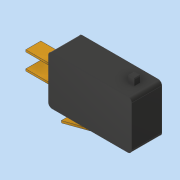
# Autodesk Inventor part: LIMIT SWITCH
Saved by Autodesk Inventor 2017 (Build 210142000, 142)
## iProperties
Created: 2016-02-15
Part Number: LIMIT SWITCH
Material: Generic
Document SubType Name: Modeling
Designer: techn
Density: 1 g/cm^3
Appearance: Smooth - Black
Author: techn
Autodesk Inventor part; units mm, degrees
ref_plane "YZ Plane" through (0, 0, 0) normal (1, 0, 0) x (0, 1, 0)
ref_plane "XZ Plane" through (0, 0, 0) normal (0, 1, 0) x (-1, 0, 0)
ref_plane "XY Plane" through (0, 0, 0) normal (0, 0, 1) x (1, 0, 0)
sketch "Sketch1" plane through (0, 0, 0) normal (0, 0, 1) x (1, 0, 0)
  line L0 (0, 0) -> (27.94, 0)
  line L1 (27.94, 0) -> (27.94, 16.256)
  line L2 (27.94, 16.256) -> (0, 16.256)
  line L3 (0, 16.256) -> (0, 0)
  dimension "d0" = 27.94
  dimension "d1" = 16.256
  constraints: 8 end point, 2 parallel, 1 horizontal, 1 perpendicular
  measures "d0" distance of L2.end L1.end
  measures "d1" distance of L1.end L0.end
extrude "Extrusion1" add sketch "Sketch1" along normal blind 10.16
fillet "Fillet1" radius 1.27 4 edges at (0, 16.256, 5.08) (27.94, 16.256, 5.08) (27.94, 0, 5.08) (0, 0, 5.08)
sketch "Sketch3" plane through (0, 0, 10.16) normal (0, 0, 1) x (1, 0, 0)
  arc A0 (0, 1.27) -> (1.27, 0) centre (1.27, 1.27) ccw projected
  line L0 (1.27, 0) -> (26.67, 0) projected
  arc A1 (26.67, 0) -> (27.94, 1.27) centre (26.67, 1.27) ccw projected
  line L1 (27.94, 1.27) -> (27.94, 14.986) projected
  arc A2 (27.94, 14.986) -> (26.67, 16.256) centre (26.67, 14.986) ccw projected
  line L2 (26.67, 16.256) -> (1.27, 16.256) projected
  arc A3 (1.27, 16.256) -> (0, 14.986) centre (1.27, 14.986) ccw projected
  line L3 (0, 14.986) -> (0, 1.27) projected
  line L4 (26.67, 16.256) -> (1.27, 16.256) projected
  line L5 (24.765, 16.256) -> (24.765, 18.542)
  line L6 (24.765, 18.542) -> (22.733, 18.542)
  line L7 (22.733, 18.542) -> (22.733, 16.256)
  point P0 (0, 0)
  dimension "d12" = 2.286
  dimension "d13" = 2.032
  dimension "d14" = 3.175
  constraints: 6 end point, 2 perpendicular, 2 point on line, 1 horizontal
  measures "d12" distance of L5.start L5.end
  measures "d13" distance of L5.end L6.end
  measures "d14" distance between parallel lines of L1 L5
ref_plane "Work Plane1" through (0, 0, 5.08) normal (0, 0, 1) x (1, 0, 0)
sketch "Sketch4" plane through (0, 0, 5.08) normal (0, 0, 1) x (1, 0, 0)
  line L0 (24.765, 18.542) -> (22.733, 18.542) projected
  line L1 (22.733, 18.542) -> (22.733, 16.256) projected
  line L2 (24.765, 16.256) -> (24.765, 18.542) projected
  line L3 (22.733, 16.256) -> (24.765, 16.256)
  line L4 (26.67, 16.256) -> (1.27, 16.256) projected
  point P0 (0, 0)
  constraints: 2 end point, 1 collinear
extrude "Extrusion3" add sketch "Sketch4" along normal mid plane 2.032
fillet "Fillet2" radius 0.254 2 edges at (24.765, 18.542, 5.08) (22.733, 18.542, 5.08)
ref_plane "Work Plane2" through (0, 0, 7.62) normal (0, 0, 1) x (1, 0, 0)
sketch "Sketch5" plane through (0, 0, 7.62) normal (0, 0, 1) x (1, 0, 0)
  arc A0 (0, 1.27) -> (1.27, 0) centre (1.27, 1.27) ccw projected
  line L0 (1.27, 0) -> (26.67, 0) projected
  arc A1 (26.67, 0) -> (27.94, 1.27) centre (26.67, 1.27) ccw projected
  line L1 (27.94, 1.27) -> (27.94, 14.986) projected
  arc A2 (27.94, 14.986) -> (26.67, 16.256) centre (26.67, 14.986) ccw projected
  line L2 (26.67, 16.256) -> (1.27, 16.256) projected
  arc A3 (1.27, 16.256) -> (0, 14.986) centre (1.27, 14.986) ccw projected
  line L3 (0, 14.986) -> (0, 1.27) projected
  line L4 (0, 14.986) -> (0, 1.27) projected
  line L5 (0, 10.1931) -> (-10.16, 10.1931)
  line L6 (-10.16, 10.1931) -> (-10.16, 9.5581)
  line L7 (-10.16, 9.5581) -> (0, 9.5581)
  line L8 (0, 9.5581) -> (0, 10.1931)
  line L9 (0, 4.6288) -> (-10.16, 4.6288)
  line L10 (-10.16, 4.6288) -> (-10.16, 3.9938)
  line L11 (-10.16, 3.9938) -> (0, 3.9938)
  line L12 (0, 3.9938) -> (0, 4.6288)
  line L13 (11.4462, 0) -> (10.8112, 0)
  line L14 (10.8112, 0) -> (10.8112, -2.1198)
  line L15 (10.8112, -2.1198) -> (11.4462, -2.1198)
  line L16 (11.4462, -2.1198) -> (11.4462, 0)
  line L17 (10.8112, -2.1198) -> (1.7523, -4.475)
  line L18 (1.7523, -4.475) -> (1.912, -5.0896)
  line L19 (1.912, -5.0896) -> (11.4462, -2.6109)
  line L20 (11.4462, -2.6109) -> (11.4462, -2.1198)
  point P0 (0, 0)
  dimension "d19" = 10.16
  dimension "d20" = 0.635
  dimension "d21" = 0.635
  dimension "d22" = 0.635
  constraints: 32 end point, 7 parallel, 4 perpendicular, 4 point on line, 3 horizontal, 1 collinear, 1 vertical
  measures "d19" distance of L5.start L5.end
  measures "d20" distance of L5.end L6.end
  measures "d21" distance of L15.end L14.end
  measures "d22" distance of L17.end L18.end
extrude "Extrusion4" add sketch "Sketch5" against normal blind 5.08 contours L11 L10 L9 L3 | L0 L16 L15 L14 | L15 L20 L19 L18 L17 | L7 L6 L5 L3
body "Solid1"
